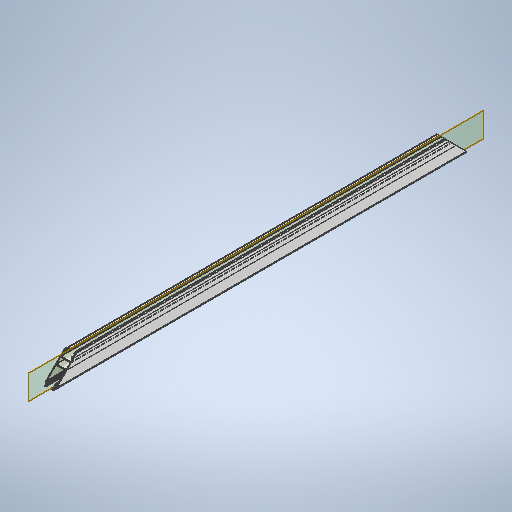
# Autodesk Inventor part: SP40-10 HOJA CORREDERA 1131 mm
Saved by Autodesk Inventor 2025 (Build 290162000, 162)
## iProperties
Created: 2026-01-18
Part Number: SP40-10 HOJA CORREDERA 1131 mm
Material: Aluminio
Document SubType Name: Modeling
Designer: ROLANDO
Density: 2.7 g/cm^3
Appearance: Satinado
Author: ROLANDO
Autodesk Inventor part; units mm, degrees
ref_plane "YZ Plane" through (0, 0, 0) normal (1, 0, 0) x (0, 1, 0)
ref_plane "XZ Plane" through (0, 0, 0) normal (0, 1, 0) x (-1, 0, 0)
sketch "Boceto1" plane through (0, 0, 0) normal (0, 0, 1) x (1, 0, 0)
  line L0 (28.1307, 40.0149) -> (1.9307, 40.0149)
  line L1 (1.9307, 41.4149) -> (28.1307, 41.4149)
  line L2 (0.0307, -0.1851) -> (0.0307, 51.6749)
  line L3 (24.8307, 55.8149) -> (24.8307, 54.1749)
  line L4 (28.6307, 54.4149) -> (28.6307, 47.9149)
  line L5 (28.6307, 46.5149) -> (24.8307, 46.5149)
  line L6 (24.8307, 46.5149) -> (24.8307, 48.1549)
  line L7 (26.2307, 47.9149) -> (28.6307, 47.9149)
  line L8 (26.2307, 49.1649) -> (25.5249, 49.1649)
  line L9 (25.5249, 49.1649) -> (24.8307, 48.1549)
  line L10 (26.2307, 53.1649) -> (25.5249, 53.1649)
  line L11 (1.4307, 41.9149) -> (1.4307, 48.9149)
  line L12 (1.4307, 48.9149) -> (2.9307, 48.9149)
  line L13 (2.9307, 48.9149) -> (2.9307, 51.6749)
  line L14 (4.1707, 55.8149) -> (10.8307, 55.8149)
  line L15 (9.3926, 54.4149) -> (5.6707, 54.4149)
  line L16 (10.8307, 55.8149) -> (10.8307, 53.3149)
  line L17 (10.8307, 53.3149) -> (10.1207, 53.3149)
  line L18 (10.1207, 53.3149) -> (9.3926, 54.4149)
  line L19 (26.2307, 54.4149) -> (28.6307, 54.4149)
  arc A0 (5.6707, 54.4149) -> (2.9307, 51.6749) centre (5.6707, 51.6749) ccw
  arc A1 (4.1707, 55.8149) -> (0.0307, 51.6749) centre (4.1707, 51.6749) ccw
  line L20 (24.8307, 54.1749) -> (25.5249, 53.1649)
  line L21 (26.2307, 54.4149) -> (26.2307, 53.1649)
  line L22 (26.2307, 47.9149) -> (26.2307, 49.1649)
  arc A2 (1.9307, 40.0149) -> (1.4307, 39.5149) centre (1.9307, 39.5149) ccw
  arc A3 (28.6307, 39.5149) -> (28.1307, 40.0149) centre (28.1307, 39.5149) ccw
  arc A4 (28.1307, 41.4149) -> (28.6307, 41.9149) centre (28.1307, 41.9149) ccw
  arc A5 (1.4307, 41.9149) -> (1.9307, 41.4149) centre (1.9307, 41.9149) ccw
  line L23 (30.0307, 55.8149) -> (24.8307, 55.8149)
  line L24 (28.6307, 41.9149) -> (28.6307, 46.5149)
  line L25 (30.0307, 55.8149) -> (30.0307, -0.1851)
  line L26 (1.4307, 29.0149) -> (28.6307, 29.0149)
  line L27 (1.4307, 27.6149) -> (28.6307, 27.6149)
  line L28 (1.4307, 39.5149) -> (1.4307, 29.0149)
  line L29 (1.4307, 27.6149) -> (1.4307, 1.2149)
  line L30 (28.6307, 1.2149) -> (28.6307, 27.6149)
  line L31 (28.6307, 29.0149) -> (28.6307, 39.5149)
  line L32 (28.6307, 39.5149) -> (28.6307, 29.0149)
  line L33 (28.6307, 27.6149) -> (28.6307, 1.2149)
  line L34 (4.5307, 5.9149) -> (6.8307, 5.9149)
  line L35 (7.8307, 4.9149) -> (7.8307, 2.5149)
  line L36 (7.8307, 2.5149) -> (6.4307, 2.5149)
  line L37 (6.4307, 2.5149) -> (6.4307, 4.5149)
  line L38 (6.4307, 4.5149) -> (4.9307, 4.5149)
  line L39 (4.9307, 4.5149) -> (4.9307, -3.4851)
  line L40 (4.9307, -3.4851) -> (6.4307, -3.4851)
  line L41 (6.4307, -3.4851) -> (6.4307, -1.4851)
  line L42 (6.4307, -1.4851) -> (7.8307, -1.4851)
  line L43 (7.8307, -1.4851) -> (7.8307, -3.8851)
  line L44 (6.8307, -4.8851) -> (3.5307, -4.8851)
  line L45 (3.5307, -4.8851) -> (3.5307, -0.1851)
  arc A6 (7.8307, 4.9149) -> (6.8307, 5.9149) centre (6.8307, 4.9149) ccw
  arc A7 (4.5307, 5.9149) -> (3.5307, 4.9149) centre (4.5307, 4.9149) ccw
  arc A8 (6.8307, -4.8851) -> (7.8307, -3.8851) centre (6.8307, -3.8851) ccw
  line L46 (3.5307, 1.2149) -> (1.4307, 1.2149)
  line L47 (3.5307, -0.1851) -> (0.0307, -0.1851)
  line L48 (3.5307, 1.2149) -> (3.5307, 4.9149)
  line L49 (25.5307, 5.9149) -> (23.2307, 5.9149)
  line L50 (22.2307, 4.9149) -> (22.2307, 2.5149)
  line L51 (22.2307, 2.5149) -> (23.6307, 2.5149)
  line L52 (23.6307, 2.5149) -> (23.6307, 4.5149)
  line L53 (23.6307, 4.5149) -> (25.1307, 4.5149)
  line L54 (25.1307, 4.5149) -> (25.1307, -3.4851)
  line L55 (25.1307, -3.4851) -> (23.6307, -3.4851)
  line L56 (23.6307, -3.4851) -> (23.6307, -1.4851)
  line L57 (23.6307, -1.4851) -> (22.2307, -1.4851)
  line L58 (22.2307, -1.4851) -> (22.2307, -3.8851)
  line L59 (23.2307, -4.8851) -> (26.5307, -4.8851)
  line L60 (26.5307, -4.8851) -> (26.5307, -0.1851)
  arc A9 (23.2307, 5.9149) -> (22.2307, 4.9149) centre (23.2307, 4.9149) ccw
  arc A10 (26.5307, 4.9149) -> (25.5307, 5.9149) centre (25.5307, 4.9149) ccw
  arc A11 (22.2307, -3.8851) -> (23.2307, -4.8851) centre (23.2307, -3.8851) ccw
  line L61 (26.5307, 1.2149) -> (28.6307, 1.2149)
  line L62 (26.5307, -0.1851) -> (30.0307, -0.1851)
  line L63 (26.5307, 1.2149) -> (26.5307, 4.9149)
  point P0 (28.6307, 51.1649)
  point P1 (0.0307, 0.7149)
  point P2 (4.9307, 0.5149)
  point P3 (25.1307, 0.5149)
  dimension "d31" = 1.4
  dimension "d42" = 2.5
  dimension "d43" = 0.71
  dimension "d45" = 2.9
  dimension "d47" = 33.5
  dimension "d48" = 7.5
  dimension "d51" = 2.74
  dimension "d59" = 6.9
  dimension "d60" = 1.4
  dimension "d78" = 6.5
  dimension "d84" = 1.4
  dimension "d85" = 1.4
  dimension "d88" = 2.4
  dimension "d95" = 6.02
  dimension "d99" = 111
  dimension "d100" = 2.4
  dimension "d108" = 4
  dimension "d109" = 0.7058
  dimension "d110" = 0.7058
  dimension "d143" = 1.4
  dimension "d147" = 1.4
  dimension "d148" = 30
  dimension "d149" = 1.4
  dimension "d150" = 14
  dimension "d151" = 27.2
  dimension "d152" = 14.4
  dimension "d153" = 1.4
  dimension "d154" = 11
  dimension "d155" = 1.4
  dimension "d156" = 1.4
  dimension "d157" = 1.4
  dimension "d158" = 1.4
  dimension "d162" = 60.7
  dimension "d163" = 10.8
  dimension "d164" = 8
  dimension "d165" = 2
  dimension "d166" = 4
  dimension "d167" = 1.5
  dimension "d168" = 7.8
  dimension "d169" = 1
  dimension "d172" = 1.4
  dimension "d173" = 4.7
  dimension "d175" = 56
  dimension "d176" = 13.8
  dimension "d177" = 14.4
  dimension "d180" = 1.5
  dimension "d181" = 4.14
  dimension "d182" = 10.8
  dimension "d183" = 14.4
  dimension "d184" = 0.5
  dimension "d187" = 3.5
  dimension "d188" = 4.9
  dimension "d189" = 6.4
  dimension "d190" = 7.8
  dimension "d191" = 26.5
  dimension "d193" = 54.6
  dimension "d195" = 3.5
  dimension "d196" = 4.9
  dimension "d197" = 53.9
  dimension "d198" = 53.7
  dimension "d202" = 2
  dimension "d203" = 3.01
  dimension "d204" = 2
  dimension "d205" = 9.3
  constraints: 128 end point, 29 tangent, 24 point on circle, 21 perpendicular, 13 parallel, 12 centre point, 12 collinear, 8 equal radius, 7 horizontal, 4 point on line, 4 vertical, 2 equal length, 2 midpoint
  measures "d31" distance between parallel lines of L15 L14
  measures "d42" distance of L14.end L16.end
  measures "d43" distance of L16.end L17.end
  measures "d45" distance between parallel lines of L13 L2
  measures "d47" angle of L16 L18
  measures "d48" distance between parallel lines of L1 L12
  measures "d51" radius of A0
  measures "d59" distance between parallel lines of L12 L14
  measures "d60" distance between parallel lines of L2 L11
  measures "d78" distance between parallel lines of L7 L19
  measures "d84" distance between parallel lines of L6 L22
  measures "d85" distance between parallel lines of L3 L21
  measures "d88" distance between parallel lines of L4 L21
  measures "d95" distance of L6.end L3.end
  measures "d99" angle of L9 L20
  measures "d100" distance between parallel lines of L4 L22
  measures "d108" distance between parallel lines of L8 L10
  measures "d109" distance of L10.start L10.end
  measures "d110" distance of L8.start L8.end
  measures "d143" distance between parallel lines of L1 L0
  measures "d147" distance between parallel lines of L7 L5
  measures "d148" distance between parallel lines of L25 L2
  measures "d149" distance between parallel lines of L25 L24
  measures "d150" distance between parallel lines of L3 L16
  measures "d151" distance between parallel lines of L4 L11
  measures "d152" distance between parallel lines of L1 L14
  measures "d153" distance between parallel lines of L27 L26
  measures "d154" distance between parallel lines of L26 L0
  measures "d155" distance between parallel lines of L35 L37
  measures "d156" distance between parallel lines of L34 L38
  measures "d157" distance between parallel lines of L43 L41
  measures "d158" distance between parallel lines of L44 L40
  measures "d162" distance between parallel lines of L44 L14
  measures "d163" distance between parallel lines of L44 L34
  measures "d164" distance between parallel lines of L40 L38
  measures "d165" distance from line of L36 point (4.931, 0.515)
  measures "d166" distance between parallel lines of L42 L36
  measures "d167" distance between parallel lines of L39 L37
  measures "d168" distance between parallel lines of L2 L43
  measures "d169" radius of A6
  measures "d172" distance between parallel lines of L46 L47
  measures "d173" distance between parallel lines of L34 L46
  measures "d175" distance between parallel lines of L14 L47
  measures "d176" distance between parallel lines of L27 L1
  measures "d177" distance between parallel lines of L23 L1
  measures "d180" distance of A0.centre A1.centre
  measures "d181" radius of A1
  measures "d182" distance between parallel lines of L16 L2
  measures "d183" distance between parallel lines of L58 L43
  measures "d184" radius of A4
  measures "d187" distance between parallel lines of L63 L25
  measures "d188" distance between parallel lines of L54 L25
  measures "d189" distance between parallel lines of L52 L25
  measures "d190" distance between parallel lines of L50 L25
  measures "d191" distance between parallel lines of L45 L25
  measures "d193" distance between parallel lines of L19 L62
  measures "d195" distance from line of L23.start L60
  measures "d196" distance from line of point (25.131, 0.515) L25
  measures "d197" distance from line of point (25.131, 0.515) L19
  measures "d198" distance from line of point (0.031, 0.715) L19
  measures "d202" distance from line of point (28.631, 51.165) L10
  measures "d203" vertical distance of point (28.631, 51.165) L3.end
  measures "d204" distance from line of point (28.631, 51.165) L8
  measures "d205" distance between parallel lines of L5 L23
extrude "Extrusión1" add sketch "Boceto1" against normal blind 1131
ref_plane "Plano de trabajo1" through (0, 0, -565.5) normal (0, 0, 1) x (1, 0, 0)
sketch "Boceto2" plane through (30.0307, -0.1851, 0) normal (1, 0, 0) x (0, 0, -1)
  line L0 (0, -4.7) -> (0, 0) projected
  line L1 (0, -4.7) -> (1131, -4.7) projected
  line L2 (1131, 0) -> (1131, -4.7) projected
  line L3 (0, 0) -> (1131, 0) projected
  line L4 (0, 0) -> (0, 56) projected
  line L5 (0, 0) -> (1131, 0) projected
  line L6 (1131, 56) -> (1131, 0) projected
  line L7 (0, 56) -> (1131, 56) projected
  line L8 (0, -4.7) -> (60.7, 56)
  line L9 (0, 56) -> (60.7, 56)
  line L10 (0, 56) -> (0, -4.7)
  point P0 (0, 0.1851)
  point P1 (0, 0)
  dimension "d201" = 45
  constraints: 6 end point, 1 collinear, 1 point on line
  measures "d201" angle of L4 L8
extrude "Extrusión2" cut sketch "Boceto2" against normal through all contours L0 L3 L8 | L4 L7 L8 L3
mirror "Simetría1" about plane through (0, 0, -565.5) normal (0, 0, 1) of "Extrusión2"
ref_plane "Plano de trabajo2" through (15.0307, -0.1851, -1126.3) normal (-1, 0, 0) x (0, 0, 1)
